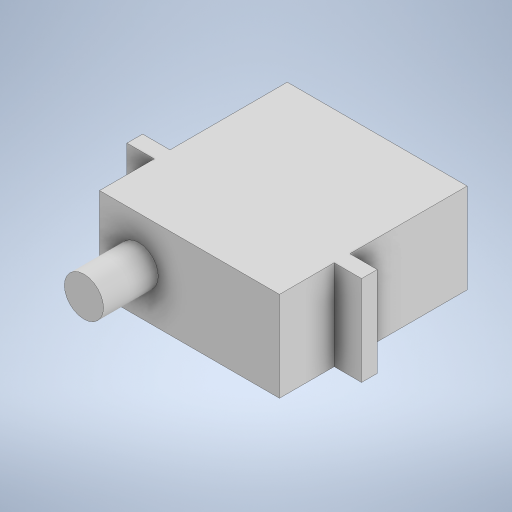
# Autodesk Inventor part: AilServoRep
Saved by Autodesk Inventor 2024.3 (Build 283343000, 343)
## iProperties
Created: 2025-01-11
Part Number: AilServoRep
Material: Generic
Document SubType Name: Modeling
Designer: jjrwe
Density: 1 g/cm^3
Appearance: Default
Author: jjrwe
Autodesk Inventor part; units mm, degrees
ref_plane "YZ Plane" through (0, 0, 0) normal (1, 0, 0) x (0, 1, 0)
ref_plane "XZ Plane" through (0, 0, 0) normal (0, 1, 0) x (-1, 0, 0)
ref_plane "XY Plane" through (0, 0, 0) normal (0, 0, 1) x (1, 0, 0)
sketch "Sketch1" plane through (0, 0, 0) normal (0, 0, 1) x (1, 0, 0)
  line L0 (0, 0) -> (23, 0)
  line L1 (23, 0) -> (23, 11.5)
  line L2 (23, 11.5) -> (0, 11.5)
  line L3 (0, 11.5) -> (0, 0)
  dimension "d0" = 23
  dimension "d1" = 11.5
  constraints: 8 end point, 2 parallel, 1 horizontal, 1 perpendicular
  measures "d0" distance of L2.end L1.end
  measures "d1" distance of L1.end L0.end
extrude "Extrusion1" add sketch "Sketch1" along normal blind 15
sketch "Sketch2" plane through (0, 0, 15) normal (0, 0, 1) x (1, 0, 0)
  line L0 (23, 11.5) -> (0, 11.5) projected
  line L1 (0, 11.5) -> (-3.5, 11.5)
  line L2 (-3.5, 11.5) -> (26.5, 11.5)
  line L3 (26.5, 11.5) -> (26.5, 0)
  line L4 (26.5, 0) -> (-3.5, 0)
  line L5 (-3.5, 0) -> (-3.5, 11.5)
  point P0 (0, 0)
  dimension "d4" = 3.5
  dimension "d5" = 30
  constraints: 10 end point, 2 horizontal, 2 parallel, 1 perpendicular
  measures "d4" distance of L0.end L1.end
  measures "d5" distance of L3.end L4.end
extrude "Extrusion2" add sketch "Sketch2" along normal blind 2
sketch "Sketch3" plane through (0, 0, 17) normal (0, 0, 1) x (1, 0, 0)
  line L0 (0, 11.5) -> (0, 0) projected
  line L1 (23, 0) -> (23, 11.5) projected
  line L2 (0, 11.5) -> (23, 11.5)
  line L3 (23, 11.5) -> (23, 0)
  line L4 (23, 0) -> (0, 0)
  line L5 (0, 0) -> (0, 11.5)
  constraints: 8 end point, 2 parallel, 1 horizontal, 1 perpendicular
extrude "Extrusion3" add sketch "Sketch3" along normal blind 7
sketch "Sketch4" plane through (0, 0, 24) normal (0, 0, 1) x (1, 0, 0)
  line L0 (0, 11.5) -> (0, 0) projected
  line L1 (0, 5.75) -> (5, 5.75)
  circle A0 centre (5, 5.75) radius 2.5
  dimension "d10" = 5
  dimension "d11" = 5
  constraints: 2 end point, 1 centre point, 1 coincident, 1 horizontal, 1 midpoint
  measures "d10" distance of L1.start L1.end
  measures "d11" diameter of A0
extrude "Extrusion4" add sketch "Sketch4" along normal blind 7
body "Solid1"
